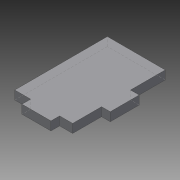
# Autodesk Inventor part: Board holders
Saved by Autodesk Inventor 2015 (Build 190159000, 159)
## iProperties
Created: 2014-11-13
Part Number: Board holders
Material: Generic
Document SubType Name: Modeling
Designer: karl
Density: 1 g/cm^3
Appearance: Default
Author: karl
Autodesk Inventor part; units mm, degrees
ref_plane "YZ Plane" through (0, 0, 0) normal (1, 0, 0) x (0, 1, 0)
ref_plane "XZ Plane" through (0, 0, 0) normal (0, 1, 0) x (-1, 0, 0)
ref_plane "XY Plane" through (0, 0, 0) normal (0, 0, 1) x (1, 0, 0)
sketch "Sketch1" plane through (0, 0, 0) normal (0, 0, 1) x (1, 0, 0)
  line L0 (-10, -16) -> (10, -16)
  line L1 (10, -16) -> (10, 16)
  line L2 (10, 16) -> (-10, 16)
  line L3 (-10, 16) -> (-10, -16)
  line L4 (-10, -16) -> (10, 16) construction
  line L5 (10, -16) -> (-10, 16) construction
  point P0 (0, 0)
  dimension "d0" = 32
  dimension "d1" = 20
  constraints: 12 end point, 2 midpoint, 2 parallel, 1 horizontal, 1 perpendicular
  measures "d0" distance of L1.end L0.end
  measures "d1" distance of L1.end L2.end
extrude "Extrusion1" add sketch "Sketch1" along normal blind 3
sketch "Sketch2" plane through (0, 0, 0) normal (0, 0, -1) x (-1, 0, 0)
  line L0 (10, -16) -> (-10, -16) projected
  line L1 (-5.5, -16) -> (4.5, -16)
  line L2 (4.5, -16) -> (4.5, -19)
  line L3 (4.5, -19) -> (-5.5, -19)
  line L4 (-5.5, -19) -> (-5.5, -16)
  line L5 (-10, -16) -> (-10, 16) projected
  point P0 (0, 0)
  dimension "d4" = 10
  dimension "d5" = 3
  dimension "d6" = 4.5
  constraints: 8 end point, 2 parallel, 1 horizontal, 1 perpendicular, 1 point on line
  measures "d4" distance of L2.end L3.end
  measures "d5" distance of L1.end L2.end
  measures "d6" distance between parallel lines of L5 L4
extrude "Extrusion2" add sketch "Sketch2" against normal blind 3
sketch "Sketch3" plane through (0, 0, 0) normal (0, 0, -1) x (-1, 0, 0)
  line L0 (-10, -16) -> (-10, 16) projected
  line L1 (-10, -6) -> (-13, -6)
  line L2 (-13, -6) -> (-13, 4)
  line L3 (-13, 4) -> (-10, 4)
  line L4 (-10, 4) -> (-10, -6)
  line L5 (-5.5, -16) -> (-10, -16) projected
  point P0 (0, 0)
  dimension "d9" = 3
  dimension "d10" = 10
  dimension "d11" = 10
  constraints: 8 end point, 2 parallel, 1 horizontal, 1 perpendicular, 1 point on line
  measures "d9" distance of L2.end L3.end
  measures "d10" distance of L1.end L2.end
  measures "d11" distance between parallel lines of L1 L5
extrude "Extrusion3" add sketch "Sketch3" against normal blind 3
sketch "Sketch4" plane through (0, 0, 0) normal (0, 0, -1) x (-1, 0, 0)
  line L0 (10, 16) -> (10, -16) projected
  line L1 (10, -3.5) -> (0, -3.5)
  line L2 (0, -3.5) -> (0, -7)
  line L3 (0, -7) -> (10, -7)
  line L4 (10, -7) -> (10, -3.5)
  line L5 (10, -16) -> (4.5, -16) projected
  point P0 (0, 0)
  dimension "d14" = 10
  dimension "d15" = 3.5
  dimension "d16" = 9
  constraints: 8 end point, 2 parallel, 1 horizontal, 1 perpendicular, 1 point on line
  measures "d14" distance of L3.end L2.end
  measures "d15" distance of L2.end L1.end
  measures "d16" distance between parallel lines of L5 L3
extrude "Extrusion4" cut sketch "Sketch4" against normal blind 3
sketch "Sketch5" plane through (0, 0, 3) normal (0, 0, 1) x (1, 0, 0)
  line L0 (10, 16) -> (-10, 16) projected
  line L1 (5.5, 16) -> (-4.5, 16)
  line L2 (-4.5, 16) -> (-4.5, 19)
  line L3 (-4.5, 19) -> (5.5, 19)
  line L4 (5.5, 19) -> (5.5, 16)
  line L5 (5.5, -19) -> (5.5, -16) projected
  point P0 (0, 0)
  dimension "d19" = 10
  dimension "d20" = 3
  constraints: 8 end point, 2 parallel, 1 collinear, 1 horizontal, 1 perpendicular, 1 point on line
  measures "d19" distance of L2.end L3.end
  measures "d20" distance of L1.end L2.end
extrude "Extrusion5" add sketch "Sketch5" against normal blind 3
body "Solid1"
